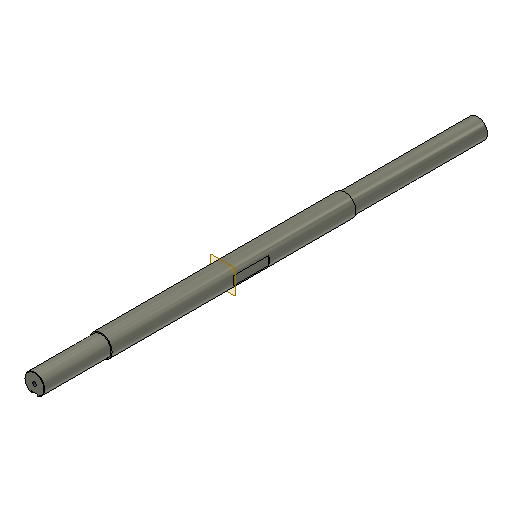
# Autodesk Inventor part: TL20240701-10110CV-013
Saved by Autodesk Inventor 2022.5 (Build 265521000, 521)
## iProperties
Category: DRIVE UNIT ASSY
Company: 현대 트랜시스(대유)
Created: 2023-04-10
Part Number: TL20240701-10110CV-013
Checked By: 김형민
Engr Approved By: 김시현
User Status: 1 x18
Material: S45C
Description: 0
Document SubType Name: Modeling
Mfg Approved By: 호상태
Designer: 박성규
Stock Number: 013
Density: 7.87 g/cm^3
Appearance: Plating Kanizen
Project: SW PJT
DETAIL: Coveryor Assembly
M/C TITLE: CJ 제일제당 협동로봇 포장시스탬 PILOT 장비
PARTS NAME: Bracket
SPECIFICATION: TA20221101-CV200000-015
DocNumber: 221118_Standard_v1
Folder: .\
VDS_Category: 엔지니어링
Detail Description: Processed products
Title: SHAFT
Subject: SW차종 시트조립라인
Author: 박성규
Revision Number: A
Autodesk Inventor part; units mm, degrees
ref_plane "YZ Plane" through (0, 0, 0) normal (1, 0, 0) x (0, 1, 0)
ref_plane "XZ Plane" through (0, 0, 0) normal (0, 1, 0) x (-1, 0, 0)
sketch "스케치9" plane through (0, 0, 0) normal (0, 0, 1) x (1, 0, 0)
  circle A0 centre (0, 0) radius 25
  dimension "d40" = 50
  constraints: 1 centre point, 1 coincident
  measures "d40" diameter of A0
extrude "돌출4" add sketch "스케치9" along normal mid plane 549.8
sketch "스케치10" plane through (0, 0, 274.9) normal (0, 0, 1) x (1, 0, 0)
  circle A0 centre (0, 0) radius 25 construction
  circle A1 centre (0, 0) radius 22.5
  dimension "d43" = 45
  constraints: 1 centre point, 1 coincident
  measures "d43" diameter of A1
extrude "돌출5" add sketch "스케치10" along normal blind 150.2
sketch "스케치11" plane through (0, 0, 425.1) normal (0, 0, 1) x (1, 0, 0)
  circle A0 centre (0, 0) radius 22.5 construction
  constraints: 1 coincident
hole "구멍3" at (0, 0, 425.1) direction (0, 0, -1) diameter 8.376 depth 27.3 tip angle 118 thread size "M10x1.5" class "6H" standard "ISO Metric profile"
chamfer "모따기1" distance 1 angle 45 1 edges at (-22.5, 0, 425.1)
sketch "스케치12" plane through (0, 0, 425.1) normal (0, 0, 1) x (1, 0, 0)
  circle A0 centre (0, 0) radius 4.188 construction
  line L0 (7, -30.625) -> (-7, -30.625)
  line L1 (-7, -30.625) -> (-7, -17)
  line L2 (-7, -17) -> (7, -17)
  line L3 (7, -17) -> (7, -30.625)
  dimension "d56" = 14
  dimension "d57" = 7
  dimension "d58" = 17
  constraints: 8 end point, 2 parallel, 1 horizontal, 1 perpendicular
  measures "d56" distance of L0.start L0.end
  measures "d57" distance from line of L1 A0.centre
  measures "d58" distance from line of L2 A0.centre
extrude "돌출6" cut sketch "스케치12" against normal blind 75
fillet "모깎기2" radius 7 2 edges at (-7, -19.1917, 350.1) (7, -19.1917, 350.1)
sketch "스케치13" plane through (0, 0, -274.9) normal (0, 0, -1) x (-1, 0, 0)
  circle A0 centre (0, 0) radius 25 construction
  circle A1 centre (0, 0) radius 22.5
  dimension "d62" = 45
  constraints: 1 centre point, 1 coincident
  measures "d62" diameter of A1
extrude "돌출7" add sketch "스케치13" along normal blind 299.2
sketch "스케치14" plane through (0, 0, -574.1) normal (0, 0, -1) x (-1, 0, 0)
  circle A0 centre (0, 0) radius 22.5 construction
  line L0 (7, -17) -> (-7, -17)
  line L1 (-7, -17) -> (-7, -32)
  line L2 (-7, -32) -> (7, -32)
  line L3 (7, -32) -> (7, -17)
  dimension "d65" = 7
  dimension "d66" = 17
  dimension "d67" = 14
  constraints: 8 end point, 2 parallel, 1 horizontal, 1 perpendicular
  measures "d65" distance from line of L1 A0.centre
  measures "d66" distance from line of A0.centre L0
  measures "d67" distance of L1.end L2.end
extrude "돌출8" cut sketch "스케치14" against normal blind 109.8
fillet "모깎기3" radius 7 2 edges at (-7, -19.1917, -464.3) (7, -19.1917, -464.3)
ref_plane "작업 평면1" through (0, 0, -304.9) normal (0, 0, -1) x (-1, 0, 0)
sketch "스케치15" plane through (0, 0, -304.9) normal (0, 0, -1) x (-1, 0, 0)
  line L0 (7, -17) -> (-7, -17)
  line L1 (-7, -17) -> (-7, -28.875)
  line L2 (-7, -28.875) -> (7, -28.875)
  line L3 (7, -28.875) -> (7, -17)
  point P0 (0, 0)
  dimension "d72" = 14
  dimension "d73" = 7
  dimension "d74" = 17
  constraints: 8 end point, 2 parallel, 1 horizontal, 1 perpendicular
  measures "d72" distance of L1.end L2.end
  measures "d73" distance from line of point (0, 0) L1
  measures "d74" distance from line of L0 point (0, 0)
extrude "돌출9" cut sketch "스케치15" along normal mid plane 55
fillet "모깎기4" radius 7 4 edges at (-7, -19.1917, -277.4) (7, -19.1917, -277.4) (7, -19.1917, -332.4) (-7, -19.1917, -332.4)
sketch "스케치16" plane through (0, 0, -574.1) normal (0, 0, -1) x (-1, 0, 0)
  arc A0 (7, -21.3834) -> (-7, -21.3834) centre (0, 0) ccw construction
  constraints: 1 coincident
hole "구멍4" at (0, 0, -574.1) direction (0, 0, 1) diameter 8.376 depth 27.3 tip angle 118 thread size "M10x1.5" class "6H" standard "ISO Metric profile"
ref_plane "Work Plane2" through (0, 0, -0.1) normal (0, 0, 1) x (1, 0, 0)
sketch "스케치17" plane through (0, 0, -0.1) normal (0, 0, 1) x (1, 0, 0)
  line L0 (-51.9353, 42.0877) -> (-23, 42.0877)
  line L1 (-23, 42.0877) -> (-23, -36.8156)
  line L2 (-23, -36.8156) -> (-51.9353, -36.8156)
  line L3 (-51.9353, -36.8156) -> (-51.9353, 42.0877)
  line L4 (23, 42.0877) -> (44.5967, 42.0877)
  line L5 (44.5967, 42.0877) -> (44.5967, -36.8156)
  line L6 (44.5967, -36.8156) -> (23, -36.8156)
  line L7 (23, -36.8156) -> (23, 42.0877)
  point P0 (0, 0)
  dimension "d85" = 23
  dimension "d86" = 23
  constraints: 16 end point, 4 parallel, 2 horizontal, 2 perpendicular, 2 point on line
  measures "d85" horizontal distance of point (0, 0) L0.end
  measures "d86" distance from line of L7 point (0, 0)
extrude "돌출10" cut sketch "스케치17" against normal blind 80
